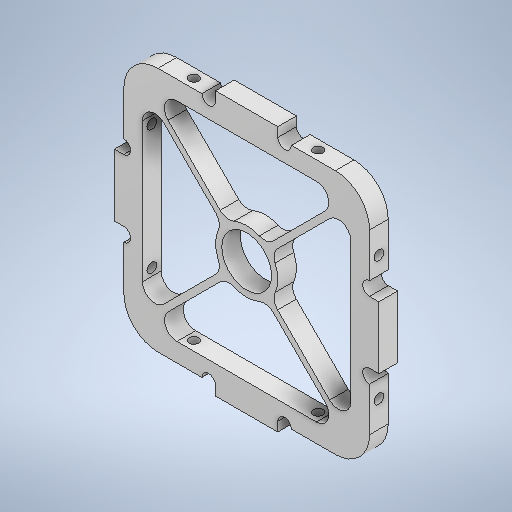
# Autodesk Inventor part: t3kata
Saved by Autodesk Inventor 2025.1 (Build 291241000, 241)
## iProperties
Created: 2024-09-04
Part Number: t3kata
Material: アルミニウム 2014-T4
Document SubType Name: Modeling
Designer: right
Density: 2.8 g/cm^3
Appearance: サテン
Mass: 4.92578 g
Surface Area: 26.5241 cm^2
Volume: 1.75921 cm^3
Author: right
Autodesk Inventor part; units mm, degrees
ref_plane "YZ Plane" through (0, 0, 0) normal (1, 0, 0) x (0, 1, 0)
ref_plane "XZ Plane" through (0, 0, 0) normal (0, 1, 0) x (-1, 0, 0)
ref_plane "XY Plane" through (0, 0, 0) normal (0, 0, 1) x (1, 0, 0)
sketch "スケッチ1" plane through (0, 0, 0) normal (0, 0, 1) x (1, 0, 0)
  line L0 (-19.75, -19.75) -> (19.75, -19.75)
  line L1 (19.75, -19.75) -> (19.75, 19.75)
  line L2 (19.75, 19.75) -> (-19.75, 19.75)
  line L3 (-19.75, 19.75) -> (-19.75, -19.75)
  line L4 (-19.75, -19.75) -> (19.75, 19.75) construction
  line L5 (19.75, -19.75) -> (-19.75, 19.75) construction
  line L6 (-5, 19.75) -> (5, 19.75)
  line L7 (5, 19.75) -> (5, 21.25)
  line L8 (5, 21.25) -> (-5, 21.25)
  line L9 (-5, 21.25) -> (-5, 19.75)
  circle A0 centre (0, 0) radius 19.75 construction
  circle A1 centre (-6.1, 19.75) radius 1.1
  line L10 (0, 21.25) -> (0, 19.75) construction
  circle A2 centre (6.1, 19.75) radius 1.1
  circle A3 centre (-19.75, -6.1) radius 1.1
  line L11 (-21.25, 5) -> (-21.25, -5)
  line L12 (-21.25, -5) -> (-19.75, -5)
  line L13 (-19.75, 5) -> (-21.25, 5)
  circle A4 centre (-19.75, 6.1) radius 1.1
  circle A5 centre (6.1, -19.75) radius 1.1
  line L14 (-5, -21.25) -> (5, -21.25)
  line L15 (5, -21.25) -> (5, -19.75)
  line L16 (-5, -19.75) -> (-5, -21.25)
  circle A6 centre (-6.1, -19.75) radius 1.1
  circle A7 centre (19.75, 6.1) radius 1.1
  line L17 (21.25, -5) -> (21.25, 5)
  line L18 (21.25, 5) -> (19.75, 5)
  line L19 (19.75, -5) -> (21.25, -5)
  circle A8 centre (19.75, -6.1) radius 1.1
  point P0 (-21.25, 0)
  point P1 (0, -21.25)
  point P2 (21.25, 0)
  point P3 (-19.75, -7.2)
  point P4 (-7.2, -19.75)
  point P5 (-5, -19.75)
  point P6 (7.2, -19.75)
  point P7 (19.75, -7.2)
  point P8 (19.75, -5)
  point P9 (19.75, 7.2)
  point P10 (7.2, 19.75)
  point P11 (5, 19.75)
  point P12 (-7.2, 19.75)
  point P13 (-19.75, 7.2)
  point P14 (-19.75, 5)
  dimension "d3" = 2.2
  dimension "d0" = 39.5
  dimension "d1" = 1.5
  dimension "d2" = 10
  dimension "d6" = 360
  constraints: 40 end point, 4 centre point, 4 midpoint, 4 parallel, 3 horizontal, 3 perpendicular, 2 point on line, 2 vertical alignment, 1 coincident, 1 symmetric about line, 64 other
  measures "d0" distance of L1.end L2.end
  measures "d1" distance between parallel lines of L2 L8
  measures "d2" distance of L7.end L8.end
extrude "押し出し1" add sketch "スケッチ1" along normal blind 3 contours A6 L0 L3 A3 A4 L2 A1 A2 L1 A7 A8 A5 | L0 L15 L14 L16 | L12 L11 L13 L3 | L1 L18 L17 L19 | L9 L8 L7 L2
sketch "スケッチ4" plane through (0, 0, 3) normal (0, 0, 1) x (1, 0, 0)
  line L0 (-16.75, -16.75) -> (16.75, -16.75)
  line L1 (16.75, -16.75) -> (16.75, 16.75)
  line L2 (16.75, 16.75) -> (-16.75, 16.75)
  line L3 (-16.75, 16.75) -> (-16.75, -16.75)
  line L4 (-16.75, -16.75) -> (16.75, 16.75) construction
  line L5 (16.75, -16.75) -> (-16.75, 16.75) construction
  arc A0 (-7.2, 19.75) -> (-5, 19.75) centre (-6.1, 19.75) ccw projected
  arc A1 (-19.75, 5) -> (-19.75, 7.2) centre (-19.75, 6.1) ccw projected
  line L6 (-7.2, 19.75) -> (-19.75, 19.75) projected
  line L7 (-19.75, 19.75) -> (-19.75, 7.2) projected
  circle A2 centre (0, 0) radius 4
  circle A3 centre (0, 0) radius 5
  line L8 (-16.0429, 16.75) -> (16.75, -16.0429)
  line L9 (-16.75, 16.0429) -> (16.0429, -16.75)
  line L10 (0, 16.75) -> (0, 0) construction
  line L11 (16.0429, 16.75) -> (-16.75, -16.0429)
  line L12 (16.75, 16.0429) -> (-16.0429, -16.75)
  point P0 (-6.1, 18.65)
  point P1 (-18.65, 6.1)
  point P2 (-3.1643, -3.8714)
  point P3 (-16.0429, -16.75)
  point P4 (3.1643, -3.8714)
  point P5 (16.75, 16.0429)
  point P6 (3.8714, 3.1643)
  point P7 (3.8714, -3.1643)
  point P8 (-16.75, -16.0429)
  point P9 (-3.8714, -3.1643)
  point P10 (-3.8714, 3.1643)
  point P11 (-16.75, 16.0429)
  point P12 (3.1643, 3.8714)
  point P13 (16.0429, 16.75)
  point P14 (-3.1643, 3.8714)
  dimension "d30" = 3
  dimension "d31" = 3
  dimension "d32" = 8
  dimension "d33" = 10
  dimension "d34" = 0.5
  constraints: 22 end point, 6 symmetric about line, 3 midpoint, 3 parallel, 2 centre point, 2 coincident, 2 point on circle, 2 point on line, 1 horizontal, 1 perpendicular, 1 vertical
  measures "d30" distance between parallel lines of L2 L6
  measures "d31" distance between parallel lines of L7 L3
  measures "d32" diameter of A2
  measures "d33" diameter of A3
  measures "d34" distance between parallel lines of L5 L8
extrude "押し出し2" cut sketch "スケッチ4" against normal through all contours L12 A3 L9 L0 | L3 L9 A3 L11 | L12 L9 A2 | A2 L11 L9 L12 | A2 L9 L11 | L8 A3 L12 L1 | L9 L12 L8 A2 | L9 L11 L8 L12 | L2 L11 A3 L8 | A2 L8 L11 L9 | L8 L12 A2 | L8 L11 A2 L12 | A2 L11 L8
fillet "フィレット1" radius 2 16 edges at (-16.75, 16.0429, 1.5) (-16.0429, 16.75, 1.5) (16.75, 16.0429, 1.5) (16.0429, 16.75, 1.5) (16.0429, -16.75, 1.5) (16.75, -16.0429, 1.5) (-16.0429, -16.75, 1.5) (-16.75, -16.0429, 1.5) (-3.1643, -3.8714, 1.5) (3.1643, -3.8714, 1.5) (3.8714, -3.1643, 1.5) (3.8714, 3.1643, 1.5) (3.1643, 3.8714, 1.5) (-3.1643, 3.8714, 1.5) (-3.8714, 3.1643, 1.5) (-3.8714, -3.1643, 1.5)
sketch "スケッチ2" plane through (-19.75, 7.2, 0) normal (-1, 0, 0) x (0, 0, 1)
  line L0 (0, -2.2) -> (3, -2.2) projected
  line L1 (0, -12.2) -> (3, -12.2) projected
  point P0 (0, -7.2)
  point P1 (1.5, 2.8)
  point P2 (1.5, -17.2)
  point P3 (1.5, -2.2)
  point P4 (1.5, -12.2)
  point P5 (1.5, -2.2)
  point P6 (1.5, -12.2)
  dimension "d10" = 5
  dimension "d11" = 5
  constraints: 4 midpoint, 2 vertical alignment
  measures "d10" distance of point (1.5, 2.8) point (1.5, -2.2)
  measures "d11" distance of point (1.5, -17.2) point (1.5, -12.2)
hole "穴1" at (-19.75, 10, 1.5) at (-19.75, -10, 1.5) direction (1, 0, 0) diameter 1.567 end through all thread size "M2x0.4" class "6H" standard "ISO Metric profile"
sketch "スケッチ3" plane through (-19.75, 19.75, 0) normal (0, 1, 0) x (1, 0, 0)
  line L0 (14.75, 0) -> (14.75, -3) projected
  line L1 (24.75, 0) -> (24.75, -3) projected
  point P0 (19.75, 0)
  point P1 (9.75, -1.5)
  point P2 (29.75, -1.5)
  point P3 (14.75, -1.5)
  point P4 (24.75, -1.5)
  point P5 (14.75, -1.5)
  point P6 (24.75, -1.5)
  dimension "d19" = 5
  dimension "d20" = 5
  constraints: 4 midpoint, 2 horizontal alignment
  measures "d19" distance of point (14.75, -1.5) point (9.75, -1.5)
  measures "d20" distance of point (24.75, -1.5) point (29.75, -1.5)
hole "穴2" at (-10, 19.75, 1.5) at (10, 19.75, 1.5) direction (0, -1, 0) diameter 1.567 end through all thread size "M2x0.4" class "6H" standard "ISO Metric profile"
sketch "スケッチ5" plane through (0, 0, 3) normal (0, 0, 1) x (1, 0, 0)
  line L0 (-16.75, -16.75) -> (16.75, -16.75)
  line L1 (16.75, -16.75) -> (16.75, 16.75)
  line L2 (16.75, 16.75) -> (-16.75, 16.75)
  line L3 (-16.75, 16.75) -> (-16.75, -16.75)
  line L4 (-16.75, -16.75) -> (16.75, 16.75) construction
  line L5 (16.75, -16.75) -> (-16.75, 16.75) construction
  arc A0 (12.6287, 13.3358) -> (11.2145, 16.75) centre (11.2145, 14.75) ccw projected
  arc A1 (16.75, 11.2145) -> (13.3358, 12.6287) centre (14.75, 11.2145) ccw projected
  line L6 (13.3358, -12.6287) -> (4.9769, -4.2698) projected
  arc A2 (4.5651, -2.0397) -> (4.9769, -4.2698) centre (6.3911, -2.8555) ccw projected
  arc A3 (4.5651, -2.0397) -> (4.5651, 2.0397) centre (0, 0) ccw projected
  arc A4 (4.9769, 4.2698) -> (4.5651, 2.0397) centre (6.3911, 2.8555) ccw projected
  line L7 (4.9769, 4.2698) -> (13.3358, 12.6287) projected
  arc A5 (16.75, 11.2145) -> (13.3358, 12.6287) centre (14.75, 11.2145) ccw projected
  line L8 (16.75, 11.2145) -> (16.75, -11.2145) projected
  arc A6 (13.3358, -12.6287) -> (16.75, -11.2145) centre (14.75, -11.2145) ccw projected
  line L9 (4.2698, -4.9769) -> (12.6287, -13.3358) projected
  arc A7 (11.2145, -16.75) -> (12.6287, -13.3358) centre (11.2145, -14.75) ccw projected
  line L10 (11.2145, -16.75) -> (-11.2145, -16.75) projected
  arc A8 (-12.6287, -13.3358) -> (-11.2145, -16.75) centre (-11.2145, -14.75) ccw projected
  line L11 (-12.6287, -13.3358) -> (-4.2698, -4.9769) projected
  arc A9 (-2.0397, -4.5651) -> (-4.2698, -4.9769) centre (-2.8555, -6.3911) ccw projected
  arc A10 (-2.0397, -4.5651) -> (2.0397, -4.5651) centre (0, 0) ccw projected
  arc A11 (4.2698, -4.9769) -> (2.0397, -4.5651) centre (2.8555, -6.3911) ccw projected
  line L12 (-13.3358, 12.6287) -> (-4.9769, 4.2698) projected
  arc A12 (-4.5651, 2.0397) -> (-4.9769, 4.2698) centre (-6.3911, 2.8555) ccw projected
  arc A13 (-4.5651, 2.0397) -> (-4.5651, -2.0397) centre (0, 0) ccw projected
  arc A14 (-4.9769, -4.2698) -> (-4.5651, -2.0397) centre (-6.3911, -2.8555) ccw projected
  line L13 (-4.9769, -4.2698) -> (-13.3358, -12.6287) projected
  arc A15 (-16.75, -11.2145) -> (-13.3358, -12.6287) centre (-14.75, -11.2145) ccw projected
  line L14 (-16.75, -11.2145) -> (-16.75, 11.2145) projected
  arc A16 (-13.3358, 12.6287) -> (-16.75, 11.2145) centre (-14.75, 11.2145) ccw projected
  circle A17 centre (0, 0) radius 4 projected
  line L15 (-4.2698, 4.9769) -> (-12.6287, 13.3358) projected
  arc A18 (-11.2145, 16.75) -> (-12.6287, 13.3358) centre (-11.2145, 14.75) ccw projected
  line L16 (-11.2145, 16.75) -> (11.2145, 16.75) projected
  arc A19 (12.6287, 13.3358) -> (11.2145, 16.75) centre (11.2145, 14.75) ccw projected
  line L17 (12.6287, 13.3358) -> (4.2698, 4.9769) projected
  arc A20 (2.0397, 4.5651) -> (4.2698, 4.9769) centre (2.8555, 6.3911) ccw projected
  arc A21 (2.0397, 4.5651) -> (-2.0397, 4.5651) centre (0, 0) ccw projected
  arc A22 (-4.2698, 4.9769) -> (-2.0397, 4.5651) centre (-2.8555, 6.3911) ccw projected
  line L18 (-21.25, -5) -> (-19.75, -5) projected
  arc A23 (-19.75, -7.2) -> (-19.75, -5) centre (-19.75, -6.1) ccw projected
  line L19 (-19.75, -7.2) -> (-19.75, -19.75) projected
  line L20 (-19.75, -19.75) -> (-7.2, -19.75) projected
  arc A24 (-5, -19.75) -> (-7.2, -19.75) centre (-6.1, -19.75) ccw projected
  line L21 (-5, -19.75) -> (-5, -21.25) projected
  line L22 (-5, -21.25) -> (5, -21.25) projected
  line L23 (5, -21.25) -> (5, -19.75) projected
  arc A25 (7.2, -19.75) -> (5, -19.75) centre (6.1, -19.75) ccw projected
  line L24 (7.2, -19.75) -> (19.75, -19.75) projected
  line L25 (19.75, -19.75) -> (19.75, -7.2) projected
  arc A26 (19.75, -5) -> (19.75, -7.2) centre (19.75, -6.1) ccw projected
  line L26 (19.75, -5) -> (21.25, -5) projected
  line L27 (21.25, -5) -> (21.25, 5) projected
  line L28 (21.25, 5) -> (19.75, 5) projected
  arc A27 (19.75, 7.2) -> (19.75, 5) centre (19.75, 6.1) ccw projected
  line L29 (19.75, 7.2) -> (19.75, 19.75) projected
  line L30 (19.75, 19.75) -> (7.2, 19.75) projected
  arc A28 (5, 19.75) -> (7.2, 19.75) centre (6.1, 19.75) ccw projected
  line L31 (5, 19.75) -> (5, 21.25) projected
  line L32 (5, 21.25) -> (-5, 21.25) projected
  line L33 (-5, 21.25) -> (-5, 19.75) projected
  arc A29 (-7.2, 19.75) -> (-5, 19.75) centre (-6.1, 19.75) ccw projected
  line L34 (-7.2, 19.75) -> (-19.75, 19.75) projected
  line L35 (-19.75, 19.75) -> (-19.75, 7.2) projected
  arc A30 (-19.75, 5) -> (-19.75, 7.2) centre (-19.75, 6.1) ccw projected
  line L36 (-19.75, 5) -> (-21.25, 5) projected
  line L37 (-21.25, 5) -> (-21.25, -5) projected
  point P0 (11.2145, 16.75)
  point P1 (-11.2145, -16.75)
  constraints: 12 end point, 2 midpoint, 2 parallel, 2 tangent, 1 horizontal, 1 perpendicular
extrude "押し出し3" add sketch "スケッチ5" against normal up to surface (3 mm away) contours L3 A15 L13 A14 A13 A12 L12 A16 L2 A18 L15 A22 A21 A20 L17 A0 L1 A1 L7 A4 A3 A2 L6 A6 L0 A7 L9 A11 A10 A9 L11 A8
fillet "フィレット2" radius 5.5 4 edges at (-19.75, 19.75, 1.5) (19.75, 19.75, 1.5) (19.75, -19.75, 1.5) (-19.75, -19.75, 1.5)
equation "\"d31\" = d30"
equation "\"d11\" = d10"
equation "\"d20\" = d19"
